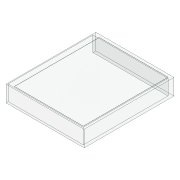
# Autodesk Inventor part: glasscover
Saved by Autodesk Inventor 2022 (Build 260153000, 153)
## iProperties
Created: 2021-06-28
Part Number: glasscover
Material: Glass
Document SubType Name: Modeling
Designer: Prajwal Patil
Density: 2.18 g/cm^3
Appearance: Clear
Author: Prajwal Patil
Autodesk Inventor part; units mm, degrees
ref_plane "YZ Plane" through (0, 0, 0) normal (1, 0, 0) x (0, 1, 0)
ref_plane "XZ Plane" through (0, 0, 0) normal (0, 1, 0) x (-1, 0, 0)
ref_plane "XY Plane" through (0, 0, 0) normal (0, 0, 1) x (1, 0, 0)
sketch "Sketch1" plane through (0, 0, 0) normal (0, 1, 0) x (-1, 0, 0)
  line L0 (14.2304, 19.7891) -> (-36.5696, 19.7891)
  line L1 (-36.5696, 19.7891) -> (-36.5696, -38.6309)
  line L2 (-36.5696, -38.6309) -> (14.2304, -38.6309)
  line L3 (14.2304, -38.6309) -> (14.2304, 19.7891)
  point P0 (0, 0)
  dimension "d0" = 50.8
  dimension "d1" = 58.42
  constraints: 8 end point, 2 parallel, 1 horizontal, 1 perpendicular
  measures "d0" distance of L2.end L1.end
  measures "d1" distance of L1.end L0.end
extrude "Extrusion1" add sketch "Sketch1" along normal blind 10.4902
sketch "Sketch2" plane through (0, 0, 0) normal (0, -1, 0) x (1, 0, 0)
  line L0 (34.5988, 18.3949) -> (-14.5151, 18.3949)
  line L1 (-14.5151, 18.3949) -> (-14.5151, -36.7441)
  line L2 (-14.5151, -36.7441) -> (34.5988, -36.7441)
  line L3 (34.5988, -36.7441) -> (34.5988, 18.3949)
  point P0 (0, 0)
  constraints: 8 end point, 2 parallel, 1 horizontal, 1 perpendicular
extrude "Extrusion2" cut sketch "Sketch2" against normal blind 9.906
sketch "Sketch3" plane through (0, 10.4902, 0) normal (0, 1, 0) x (1, 0, 0)
  line L0 (34.5988, 36.7441) -> (-14.2304, 36.7441) projected
  line L1 (-14.2304, -18.3949) -> (34.5988, -18.3949) projected
  line L2 (34.5988, 36.7441) -> (-10.1332, 36.7441)
  line L3 (-10.1332, 36.7441) -> (-10.1332, -18.3949)
  line L4 (-10.1332, -18.3949) -> (34.5988, -18.3949)
  line L5 (34.5988, -18.3949) -> (34.5988, 36.7441)
  point P0 (0, 0)
  constraints: 8 end point, 2 parallel, 1 horizontal, 1 perpendicular, 1 point on line
extrude "Extrusion3" add sketch "Sketch3" along normal blind 0.0762
body "Solid1"
